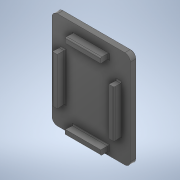
# Autodesk Inventor part: SP19V1 Tapacanto Delantero
Saved by Autodesk Inventor 2021.2 (Build 252289000, 289)
## iProperties
Created: 2026-06-08
Part Number: SP19V1 Tapacanto Delantero
Material: ABS Plastic
Document SubType Name: Modeling
Designer: NELSON
Density: 1.06 g/cm^3
Appearance: Smooth - Black
Author: NELSON
Autodesk Inventor part; units mm, degrees
ref_plane "YZ Plane" through (0, 0, 0) normal (1, 0, 0) x (0, 1, 0)
ref_plane "XZ Plane" through (0, 0, 0) normal (0, 1, 0) x (-1, 0, 0)
ref_plane "XY Plane" through (0, 0, 0) normal (0, 0, 1) x (1, 0, 0)
sketch "Boceto1" plane through (0, 0, 0) normal (0, 0, 1) x (1, 0, 0)
  line L0 (30, -40) -> (-30, -40)
  line L1 (-30, -40) -> (-30, 40)
  line L2 (-30, 40) -> (30, 40)
  line L3 (30, 40) -> (30, -40)
  line L4 (30, -40) -> (-30, 40) construction
  line L5 (-30, -40) -> (30, 40) construction
  line L6 (33.7, -43.7) -> (-33.7, -43.7)
  line L7 (-33.7, -43.7) -> (-33.7, 43.7)
  line L8 (-33.7, 43.7) -> (33.7, 43.7)
  line L9 (33.7, 43.7) -> (33.7, -43.7)
  line L10 (-33.7, -40) -> (33.7, -40)
  point P0 (0, 0)
  point P1 (30, -40)
  point P2 (-30, -40)
  dimension "d0" = 60
  dimension "d1" = 80
  dimension "d2" = 3.7
  dimension "d20" = 3.7
  constraints: 22 end point, 4 parallel, 3 perpendicular, 2 midpoint, 2 point on line, 1 horizontal, 3 other
  measures "d0" distance of L1.end L2.end
  measures "d1" distance of L0.end L1.end
  measures "d2" distance between parallel lines of L3 L9
  measures "d20" distance between parallel lines of L6 L10
extrude "Extrusión1" add sketch "Boceto1" along normal blind 5 contours L0 L1 L2 L3 | L3 L2 L1 L10 L7 L8 L9
sketch "Boceto2" plane through (0, 0, 5) normal (0, 0, 1) x (1, 0, 0)
  line L0 (-26.8, -36.8) -> (26.8, -36.8)
  line L1 (26.8, -36.8) -> (26.8, 36.8)
  line L2 (26.8, 36.8) -> (-26.8, 36.8)
  line L3 (-26.8, 36.8) -> (-26.8, -36.8)
  line L4 (-26.8, -36.8) -> (26.8, 36.8) construction
  line L5 (26.8, -36.8) -> (-26.8, 36.8) construction
  line L6 (-26.4, 36.4) -> (26.4, 36.4)
  line L7 (26.4, 36.4) -> (26.4, -36.4)
  line L8 (26.4, -36.4) -> (-26.4, -36.4)
  line L9 (-26.4, -36.4) -> (-26.4, 36.4)
  line L10 (-26.4, 0) -> (-24.4, 0)
  line L11 (-22.4, -20) -> (-26.4, -20)
  line L12 (-26.4, -20) -> (-26.4, 20)
  line L13 (-26.4, 20) -> (-22.4, 20)
  line L14 (-22.4, 20) -> (-22.4, -20)
  line L15 (-22.4, -20) -> (-26.4, 20) construction
  line L16 (-26.4, -20) -> (-22.4, 20) construction
  line L17 (0, 0) -> (0, 2.2865)
  line L18 (0, 0) -> (-0.6496, 0)
  line L19 (22.4, -20) -> (26.4, -20)
  line L20 (26.4, -20) -> (26.4, 20)
  line L21 (26.4, 20) -> (22.4, 20)
  line L22 (22.4, 20) -> (22.4, -20)
  line L23 (22.4, -20) -> (26.4, 20) construction
  line L24 (26.4, -20) -> (22.4, 20) construction
  line L25 (0, 36.4) -> (0, 34.4)
  line L26 (15, 32.4) -> (-15, 32.4)
  line L27 (-15, 32.4) -> (-15, 36.4)
  line L28 (-15, 36.4) -> (15, 36.4)
  line L29 (15, 36.4) -> (15, 32.4)
  line L30 (15, 32.4) -> (-15, 36.4) construction
  line L31 (-15, 32.4) -> (15, 36.4) construction
  line L32 (15, -32.4) -> (-15, -32.4)
  line L33 (-15, -32.4) -> (-15, -36.4)
  line L34 (-15, -36.4) -> (15, -36.4)
  line L35 (15, -36.4) -> (15, -32.4)
  line L36 (15, -32.4) -> (-15, -36.4) construction
  line L37 (-15, -32.4) -> (15, -36.4) construction
  point P0 (24.4, 0)
  point P1 (0, -34.4)
  point P2 (-15, -36.4)
  point P3 (26.4, -20)
  point P4 (26.4, 20)
  dimension "d25" = 53.6
  dimension "d26" = 73.6
  dimension "d27" = 0.4
  dimension "d28" = 2
  dimension "d29" = 40
  dimension "d30" = 2
  dimension "d31" = 30
  constraints: 76 end point, 12 midpoint, 10 symmetric about line, 8 parallel, 5 horizontal, 4 perpendicular, 2 point on line, 2 vertical, 3 other
  measures "d25" distance of L2.end L1.end
  measures "d26" distance of L1.end L0.end
  measures "d27" distance between parallel lines of L2 L6
  measures "d28" distance of L10.start L10.end
  measures "d29" distance of L11.end L12.end
  measures "d30" distance of L25.start L25.end
  measures "d31" distance of L27.end L28.end
extrude "Extrusión2" add sketch "Boceto2" along normal blind 7 draft 2 contours L6 L29 L26 L27 | L13 L14 L11 L9 | L7 L19 L22 L21 | L33 L32 L35 L8
fillet "Empalme1" radius 4.716 4 edges at (33.7, 43.7, 2.5) (-33.7, 43.7, 2.5) (33.7, -40, 2.5) (-33.7, -40, 2.5)
fillet "Empalme1" radius 1 16 edges at (0, 36.6444, 12) (26.6444, 0, 12) (0, -36.6444, 12) (-26.6444, 0, 12) (-22.4, 0, 5) (0, 32.4, 5) (0, -32.4, 5) (15, -34.4, 5) (-24.4, -20, 5) (-24.4, 20, 5) (-15, 34.4, 5) (15, 34.4, 5) (24.4, 20, 5) (24.4, -20, 5) (-15, -34.4, 5) (22.4, 0, 5)
chamfer "Chamfer1" distance 0.3 angle 45 8 edges at (0, 43.7, 0) (-32.3187, 42.3187, 0) (-33.7, 1.85, 0) (-32.3187, -38.6187, 0) (0, -40, 0) (32.3187, -38.6187, 0) (33.7, 1.85, 0) (32.3187, 42.3187, 0)
